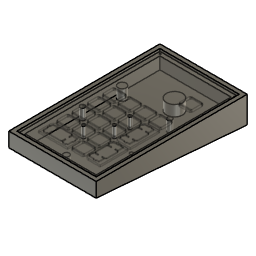
nummerical_case_+_plate (Autodesk Fusion 360 design; units mm, degrees)
Autodesk Fusion 360 part; units mm, degrees
note: some values were not read from the file. Set by a fixed rule: which sketch regions a step uses.
(part 1 of 3)
sketch "ae4adbfa673b0e7a36190fe0facbe4f336e7beb9_switch" plane through (0, 0, 0) normal (0, 0, 1) x (1, 0, 0)
  line L0 (0.0951, 148.071) -> (76.2953, 148.071)
  line L1 (76.2953, 148.071) -> (76.2953, 0.4341)
  line L2 (76.2953, 0.4341) -> (0.0951, 0.4341)
  line L3 (0.0951, 0.4341) -> (0.0951, 148.071)
  line L4 (12.1447, 16.9595) -> (12.1447, 16.3601)
  line L5 (12.1447, 16.3601) -> (11.344, 16.3601)
  line L6 (11.344, 16.3601) -> (11.344, 12.2604)
  line L7 (11.344, 12.2604) -> (10.6192, 12.2604)
  line L8 (10.6192, 12.2604) -> (10.6192, 15.4905)
  line L9 (10.6192, 15.4905) -> (3.8695, 15.4905)
  line L10 (3.8695, 15.4905) -> (3.8695, 12.2604)
  line L11 (3.8695, 12.2604) -> (3.0441, 12.2604)
  line L12 (3.0441, 12.2604) -> (3.0441, 9.4602)
  line L13 (3.0441, 9.4602) -> (3.8696, 9.4602)
  line L14 (3.8695, 9.4602) -> (3.8695, 3.1902)
  line L15 (3.8695, 3.1902) -> (5.5948, 3.1902)
  line L16 (5.5948, 3.1902) -> (5.5948, 1.9899)
  line L17 (5.5948, 1.9899) -> (8.8939, 1.9899)
  line L18 (8.8939, 1.9899) -> (8.8939, 3.1902)
  line L19 (8.8939, 3.1902) -> (10.6192, 3.1902)
  line L20 (10.6192, 3.1902) -> (10.6192, 7.6605)
  line L21 (10.6192, 7.6605) -> (11.344, 7.6605)
  line L22 (11.344, 7.6605) -> (11.344, 3.5609)
  line L23 (11.344, 3.5609) -> (12.1447, 3.5609)
  line L24 (12.1447, 3.5609) -> (12.1447, 2.96)
  line L25 (12.1447, 2.96) -> (26.1441, 2.96)
  line L26 (26.1441, 2.96) -> (26.1441, 3.5609)
  line L27 (26.1441, 3.5609) -> (26.9448, 3.5609)
  line L28 (26.9448, 3.5609) -> (26.9448, 7.6605)
  line L29 (26.9448, 7.6605) -> (27.6696, 7.6605)
  line L30 (27.6696, 7.6605) -> (27.6696, 3.1902)
  line L31 (27.6696, 3.1902) -> (29.3949, 3.1902)
  line L32 (29.3949, 3.1902) -> (29.3949, 1.9899)
  line L33 (29.3949, 1.9899) -> (32.694, 1.9899)
  line L34 (32.694, 1.9899) -> (32.694, 3.1902)
  line L35 (32.694, 3.1902) -> (34.4193, 3.1902)
  line L36 (34.4193, 3.1902) -> (34.4193, 9.4602)
  line L37 (34.4193, 9.4602) -> (35.2447, 9.4602)
  line L38 (35.2447, 9.4602) -> (35.2447, 12.2604)
  line L39 (35.2447, 12.2604) -> (34.4193, 12.2604)
  line L40 (34.4193, 12.2604) -> (34.4193, 15.4905)
  line L41 (34.4193, 15.4905) -> (27.6696, 15.4905)
  line L42 (27.6696, 15.4905) -> (27.6696, 12.2604)
  line L43 (27.6696, 12.2604) -> (26.9448, 12.2604)
  line L44 (26.9448, 12.2604) -> (26.9448, 16.3601)
  line L45 (26.9448, 16.3601) -> (26.1441, 16.3601)
  line L46 (26.1441, 16.3601) -> (26.1441, 16.9595)
  line L47 (26.1441, 16.9595) -> (12.1447, 16.9595)
  line L48 (40.7197, 16.9595) -> (40.7197, 16.3601)
  line L49 (40.7197, 16.3601) -> (39.9189, 16.3601)
  line L50 (39.9189, 16.3601) -> (39.9189, 3.5609)
  line L51 (39.9189, 3.5609) -> (40.7197, 3.5609)
  line L52 (40.7197, 3.5609) -> (40.7197, 2.96)
  line L53 (40.7197, 2.96) -> (54.719, 2.96)
  line L54 (54.719, 2.96) -> (54.719, 3.5609)
  line L55 (54.719, 3.5609) -> (55.5198, 3.5609)
  line L56 (55.5198, 3.5609) -> (55.5198, 16.3601)
  line L57 (55.5198, 16.3601) -> (54.719, 16.3601)
  line L58 (54.719, 16.3601) -> (54.719, 16.9595)
  line L59 (54.719, 16.9595) -> (40.7197, 16.9595)
  line L60 (66.27, 35.585) -> (66.27, 34.7597)
  line L61 (66.27, 34.7597) -> (59.9997, 34.7597)
  line L62 (59.9997, 34.7597) -> (59.9997, 33.0357)
  line L63 (59.9997, 33.0357) -> (58.7996, 33.0357)
  line L64 (58.7996, 33.0357) -> (58.7996, 29.7353)
  line L65 (58.7996, 29.7353) -> (59.9997, 29.7353)
  line L66 (59.9997, 29.7353) -> (59.9997, 28.01)
  line L67 (59.9997, 28.01) -> (64.4701, 28.01)
  line L68 (64.4701, 28.01) -> (64.4701, 27.2852)
  line L69 (64.4701, 27.2852) -> (60.3691, 27.2852)
  line L70 (60.3691, 27.2852) -> (60.3691, 26.4845)
  line L71 (60.3691, 26.4845) -> (59.7697, 26.4845)
  line L72 (59.7697, 26.4845) -> (59.7697, 12.485)
  line L73 (59.7697, 12.485) -> (60.3691, 12.485)
  line L74 (60.3691, 12.485) -> (60.3691, 11.6858)
  line L75 (60.3691, 11.6858) -> (64.4701, 11.6858)
  line L76 (64.4701, 11.6858) -> (64.4701, 10.9595)
  line L77 (64.4701, 10.9595) -> (59.9997, 10.9595)
  line L78 (59.9997, 10.9595) -> (59.9997, 9.2356)
  line L79 (59.9997, 9.2356) -> (58.7996, 9.2356)
  line L80 (58.7996, 9.2356) -> (58.7996, 5.9352)
  line L81 (58.7996, 5.9352) -> (59.9997, 5.9352)
  line L82 (59.9997, 5.9352) -> (59.9997, 4.2099)
  line L83 (59.9997, 4.2099) -> (66.27, 4.2099)
  line L84 (66.27, 4.2099) -> (66.27, 3.3858)
  line L85 (66.27, 3.3858) -> (69.07, 3.3858)
  line L86 (69.07, 3.3858) -> (69.07, 4.2099)
  line L87 (69.07, 4.2099) -> (72.3, 4.2099)
  line L88 (72.3, 4.2099) -> (72.3, 10.9595)
  line L89 (72.3, 10.9595) -> (69.07, 10.9595)
  line L90 (69.07, 10.9595) -> (69.07, 11.6858)
  line L91 (69.07, 11.6858) -> (73.1696, 11.6858)
  line L92 (73.1696, 11.6858) -> (73.1696, 12.485)
  line L93 (73.1696, 12.485) -> (73.769, 12.485)
  line L94 (73.769, 12.485) -> (73.769, 26.4845)
  line L95 (73.769, 26.4845) -> (73.1696, 26.4845)
  line L96 (73.1696, 26.4845) -> (73.1696, 27.2852)
  line L97 (73.1696, 27.2852) -> (69.07, 27.2852)
  line L98 (69.07, 27.2852) -> (69.07, 28.01)
  line L99 (69.07, 28.01) -> (72.3, 28.01)
  line L100 (72.3, 28.01) -> (72.3, 34.7597)
  line L101 (72.3, 34.7597) -> (69.07, 34.7597)
  line L102 (69.07, 34.7597) -> (69.07, 35.585)
  line L103 (69.07, 35.585) -> (66.27, 35.585)
  line L104 (2.6197, 36.0094) -> (2.6197, 35.4101)
  line L105 (2.6197, 35.4101) -> (1.819, 35.4101)
  line L106 (1.819, 35.4101) -> (1.819, 22.6109)
  line L107 (1.819, 22.6109) -> (2.6197, 22.6109)
  line L108 (2.6197, 22.6109) -> (2.6197, 22.01)
  line L109 (2.6197, 22.01) -> (16.6192, 22.01)
  line L110 (16.6192, 22.01) -> (16.6192, 22.6109)
  line L111 (16.6192, 22.6109) -> (17.4198, 22.6109)
  line L112 (17.4198, 22.6109) -> (17.4198, 35.4101)
  line L113 (17.4198, 35.4101) -> (16.6192, 35.4101)
  line L114 (16.6192, 35.4101) -> (16.6192, 36.0094)
  line L115 (16.6192, 36.0094) -> (2.6196, 36.0094)
  line L116 (21.6697, 36.0094) -> (21.6697, 35.4101)
  line L117 (21.6697, 35.4101) -> (20.869, 35.4101)
  line L118 (20.869, 35.4101) -> (20.869, 22.6109)
  line L119 (20.869, 22.6109) -> (21.6697, 22.6109)
  line L120 (21.6697, 22.6109) -> (21.6697, 22.01)
  line L121 (21.6697, 22.01) -> (35.669, 22.01)
  line L122 (35.669, 22.01) -> (35.669, 22.6109)
  line L123 (35.669, 22.6109) -> (36.4698, 22.6109)
  line L124 (36.4698, 22.6109) -> (36.4698, 35.4101)
  line L125 (36.4698, 35.4101) -> (35.669, 35.4101)
  line L126 (35.669, 35.4101) -> (35.669, 36.0094)
  line L127 (35.669, 36.0094) -> (21.6697, 36.0094)
  line L128 (40.7197, 36.0094) -> (40.7197, 35.4101)
  line L129 (40.7197, 35.4101) -> (39.9189, 35.4101)
  line L130 (39.9189, 35.4101) -> (39.9189, 22.6109)
  line L131 (39.9189, 22.6109) -> (40.7197, 22.6109)
  line L132 (40.7197, 22.6109) -> (40.7197, 22.01)
  line L133 (40.7197, 22.01) -> (54.719, 22.01)
  line L134 (54.719, 22.01) -> (54.719, 22.6109)
  line L135 (54.719, 22.6109) -> (55.5198, 22.6109)
  line L136 (55.5198, 22.6109) -> (55.5198, 35.4101)
  line L137 (55.5198, 35.4101) -> (54.719, 35.4101)
  line L138 (54.719, 35.4101) -> (54.719, 36.0094)
  line L139 (54.719, 36.0094) -> (40.7197, 36.0094)
  line L140 (2.6197, 55.0594) -> (2.6197, 54.4601)
  line L141 (2.6197, 54.4601) -> (1.819, 54.4601)
  line L142 (1.819, 54.4601) -> (1.819, 41.6609)
  line L143 (1.819, 41.6609) -> (2.6197, 41.6609)
  line L144 (2.6197, 41.6609) -> (2.6197, 41.0602)
  line L145 (2.6197, 41.0602) -> (16.6192, 41.0602)
  line L146 (16.6192, 41.0602) -> (16.6192, 41.6609)
  line L147 (16.6192, 41.6609) -> (17.4198, 41.6609)
  line L148 (17.4198, 41.6609) -> (17.4198, 54.4601)
  line L149 (17.4198, 54.4601) -> (16.6192, 54.4601)
  line L150 (16.6192, 54.4601) -> (16.6192, 55.0594)
  line L151 (16.6192, 55.0594) -> (2.6196, 55.0594)
  line L152 (21.6697, 55.0594) -> (21.6697, 54.4601)
  line L153 (21.6697, 54.4601) -> (20.869, 54.4601)
  line L154 (20.869, 54.4601) -> (20.869, 41.6609)
  line L155 (20.869, 41.6609) -> (21.6697, 41.6609)
  line L156 (21.6697, 41.6609) -> (21.6697, 41.0602)
  line L157 (21.6697, 41.0602) -> (35.669, 41.0602)
  line L158 (35.669, 41.0602) -> (35.669, 41.6609)
  line L159 (35.669, 41.6609) -> (36.4698, 41.6609)
  line L160 (36.4698, 41.6609) -> (36.4698, 54.4601)
  line L161 (36.4698, 54.4601) -> (35.669, 54.4601)
  line L162 (35.669, 54.4601) -> (35.669, 55.0594)
  line L163 (35.669, 55.0594) -> (21.6697, 55.0594)
  line L164 (40.7197, 55.0594) -> (40.7197, 54.4601)
  line L165 (40.7197, 54.4601) -> (39.9189, 54.4601)
  line L166 (39.9189, 54.4601) -> (39.9189, 41.6609)
  line L167 (39.9189, 41.6609) -> (40.7197, 41.6609)
  line L168 (40.7197, 41.6609) -> (40.7197, 41.0602)
  line L169 (40.7197, 41.0602) -> (54.719, 41.0602)
  line L170 (54.719, 41.0602) -> (54.719, 41.6609)
  line L171 (54.719, 41.6609) -> (55.5198, 41.6609)
  line L172 (55.5198, 41.6609) -> (55.5198, 54.4601)
  line L173 (55.5198, 54.4601) -> (54.719, 54.4601)
  line L174 (54.719, 54.4601) -> (54.719, 55.0594)
  line L175 (54.719, 55.0594) -> (40.7197, 55.0594)
  line L176 (66.27, 73.685) -> (66.27, 72.8595)
  line L177 (66.27, 72.8595) -> (59.9997, 72.8595)
  line L178 (59.9997, 72.8595) -> (59.9997, 71.1359)
  line L179 (59.9997, 71.1359) -> (58.7996, 71.1359)
  line L180 (58.7996, 71.1359) -> (58.7996, 67.8353)
  line L181 (58.7996, 67.8353) -> (59.9997, 67.8353)
  line L182 (59.9997, 67.8353) -> (59.9997, 66.1098)
  line L183 (59.9997, 66.1098) -> (64.4701, 66.1098)
  line L184 (64.4701, 66.1098) -> (64.4701, 65.3852)
  line L185 (64.4701, 65.3852) -> (60.3691, 65.3852)
  line L186 (60.3691, 65.3852) -> (60.3691, 64.5844)
  line L187 (60.3691, 64.5844) -> (59.7697, 64.5844)
  line L188 (59.7697, 64.5844) -> (59.7697, 50.5852)
  line L189 (59.7697, 50.5852) -> (60.3691, 50.5852)
  line L190 (60.3691, 50.5852) -> (60.3691, 49.7858)
  line L191 (60.3691, 49.7858) -> (64.4701, 49.7858)
  line L192 (64.4701, 49.7858) -> (64.4701, 49.0594)
  line L193 (64.4701, 49.0594) -> (59.9997, 49.0594)
  line L194 (59.9997, 49.0594) -> (59.9997, 47.3357)
  line L195 (59.9997, 47.3357) -> (58.7996, 47.3357)
  line L196 (58.7996, 47.3357) -> (58.7996, 44.0351)
  line L197 (58.7996, 44.0351) -> (59.9997, 44.0351)
  line L198 (59.9997, 44.0351) -> (59.9997, 42.31)
  line L199 (59.9997, 42.31) -> (66.27, 42.31)
  line L200 (66.27, 42.31) -> (66.27, 41.486)
  line L201 (66.27, 41.486) -> (69.07, 41.486)
  line L202 (69.07, 41.486) -> (69.07, 42.31)
  line L203 (69.07, 42.31) -> (72.3, 42.31)
  line L204 (72.3, 42.31) -> (72.3, 49.0594)
  line L205 (72.3, 49.0594) -> (69.07, 49.0594)
  line L206 (69.07, 49.0594) -> (69.07, 49.7858)
  line L207 (69.07, 49.7858) -> (73.1696, 49.7858)
  line L208 (73.1696, 49.7858) -> (73.1696, 50.5852)
  line L209 (73.1696, 50.5852) -> (73.769, 50.5852)
  line L210 (73.769, 50.5852) -> (73.769, 64.5844)
  line L211 (73.769, 64.5844) -> (73.1696, 64.5844)
  line L212 (73.1696, 64.5844) -> (73.1696, 65.3852)
  line L213 (73.1696, 65.3852) -> (69.07, 65.3852)
  line L214 (69.07, 65.3852) -> (69.07, 66.1098)
  line L215 (69.07, 66.1098) -> (72.3, 66.1098)
  line L216 (72.3, 66.1098) -> (72.3, 72.8595)
  line L217 (72.3, 72.8595) -> (69.07, 72.8595)
  line L218 (69.07, 72.8595) -> (69.07, 73.685)
  line L219 (69.07, 73.685) -> (66.27, 73.685)
  line L220 (2.6197, 74.1094) -> (2.6197, 73.5101)
  line L221 (2.6197, 73.5101) -> (1.819, 73.5101)
  line L222 (1.819, 73.5101) -> (1.819, 60.7109)
  line L223 (1.819, 60.7109) -> (2.6197, 60.7109)
  line L224 (2.6197, 60.7109) -> (2.6197, 60.1102)
  line L225 (2.6197, 60.1102) -> (16.6192, 60.1102)
  line L226 (16.6192, 60.1102) -> (16.6192, 60.7109)
  line L227 (16.6192, 60.7109) -> (17.4198, 60.7109)
  line L228 (17.4198, 60.7109) -> (17.4198, 73.5101)
  line L229 (17.4198, 73.5101) -> (16.6192, 73.5101)
  line L230 (16.6192, 73.5101) -> (16.6192, 74.1094)
  line L231 (16.6192, 74.1094) -> (2.6196, 74.1094)
  line L232 (21.6697, 74.1094) -> (21.6697, 73.5101)
  line L233 (21.6697, 73.5101) -> (20.869, 73.5101)
  line L234 (20.869, 73.5101) -> (20.869, 60.7109)
  line L235 (20.869, 60.7109) -> (21.6697, 60.7109)
  line L236 (21.6697, 60.7109) -> (21.6697, 60.1102)
  line L237 (21.6697, 60.1102) -> (35.669, 60.1102)
  line L238 (35.669, 60.1102) -> (35.669, 60.7109)
  line L239 (35.669, 60.7109) -> (36.4698, 60.7109)
  line L240 (36.4698, 60.7109) -> (36.4698, 73.5101)
  line L241 (36.4698, 73.5101) -> (35.669, 73.5101)
  line L242 (35.669, 73.5101) -> (35.669, 74.1094)
  line L243 (35.669, 74.1094) -> (21.6697, 74.1094)
  line L244 (40.7197, 74.1094) -> (40.7197, 73.5101)
  line L245 (40.7197, 73.5101) -> (39.9189, 73.5101)
  line L246 (39.9189, 73.5101) -> (39.9189, 60.7109)
  line L247 (39.9189, 60.7109) -> (40.7197, 60.7109)
  line L248 (40.7197, 60.7109) -> (40.7197, 60.1102)
  line L249 (40.7197, 60.1102) -> (54.719, 60.1102)
  line L250 (54.719, 60.1102) -> (54.719, 60.7109)
  line L251 (54.719, 60.7109) -> (55.5198, 60.7109)
  line L252 (55.5198, 60.7109) -> (55.5198, 73.5101)
  line L253 (55.5198, 73.5101) -> (54.719, 73.5101)
  line L254 (54.719, 73.5101) -> (54.719, 74.1094)
  line L255 (54.719, 74.1094) -> (40.7197, 74.1094)
  line L256 (2.6197, 93.1594) -> (2.6197, 92.5601)
  line L257 (2.6197, 92.5601) -> (1.819, 92.5601)
  line L258 (1.819, 92.5601) -> (1.819, 79.7609)
  line L259 (1.819, 79.7609) -> (2.6197, 79.7609)
  line L260 (2.6197, 79.7609) -> (2.6197, 79.1602)
  line L261 (2.6197, 79.1602) -> (16.6192, 79.1602)
  line L262 (16.6192, 79.1602) -> (16.6192, 79.7609)
  line L263 (16.6192, 79.7609) -> (17.4198, 79.7609)
  line L264 (17.4198, 79.7609) -> (17.4198, 92.5601)
  line L265 (17.4198, 92.5601) -> (16.6192, 92.5601)
  line L266 (16.6192, 92.5601) -> (16.6192, 93.1594)
  line L267 (16.6192, 93.1594) -> (2.6196, 93.1594)
  line L268 (21.6697, 93.1594) -> (21.6697, 92.5601)
  line L269 (21.6697, 92.5601) -> (20.869, 92.5601)
  line L270 (20.869, 92.5601) -> (20.869, 79.7609)
  line L271 (20.869, 79.7609) -> (21.6697, 79.7609)
  line L272 (21.6697, 79.7609) -> (21.6697, 79.1602)
  line L273 (21.6697, 79.1602) -> (35.669, 79.1602)
  line L274 (35.669, 79.1602) -> (35.669, 79.7609)
  line L275 (35.669, 79.7609) -> (36.4698, 79.7609)
  line L276 (36.4698, 79.7609) -> (36.4698, 92.5601)
  line L277 (36.4698, 92.5601) -> (35.669, 92.5601)
  line L278 (35.669, 92.5601) -> (35.669, 93.1594)
  line L279 (35.669, 93.1594) -> (21.6697, 93.1594)
  line L280 (40.7197, 93.1594) -> (40.7197, 92.5601)
  line L281 (40.7197, 92.5601) -> (39.9189, 92.5601)
  line L282 (39.9189, 92.5601) -> (39.9189, 79.7609)
  line L283 (39.9189, 79.7609) -> (40.7197, 79.7609)
  line L284 (40.7197, 79.7609) -> (40.7197, 79.1602)
  line L285 (40.7197, 79.1602) -> (54.719, 79.1602)
  line L286 (54.719, 79.1602) -> (54.719, 79.7609)
  line L287 (54.719, 79.7609) -> (55.5198, 79.7609)
  line L288 (55.5198, 79.7609) -> (55.5198, 92.5601)
  line L289 (55.5198, 92.5601) -> (54.719, 92.5601)
  line L290 (54.719, 92.5601) -> (54.719, 93.1594)
  line L291 (54.719, 93.1594) -> (40.7197, 93.1594)
  line L292 (59.7697, 93.1594) -> (59.7697, 92.5601)
  line L293 (59.7697, 92.5601) -> (58.9689, 92.5601)
  line L294 (58.9689, 92.5601) -> (58.9689, 79.7609)
  line L295 (58.9689, 79.7609) -> (59.7697, 79.7609)
  line L296 (59.7697, 79.7609) -> (59.7697, 79.1602)
  line L297 (59.7697, 79.1602) -> (73.769, 79.1602)
  line L298 (73.769, 79.1602) -> (73.769, 79.7609)
  line L299 (73.769, 79.7609) -> (74.5698, 79.7609)
  line L300 (74.5698, 79.7609) -> (74.5698, 92.5601)
  line L301 (74.5698, 92.5601) -> (73.769, 92.5601)
  line L302 (73.769, 92.5601) -> (73.769, 93.1594)
  line L303 (73.769, 93.1594) -> (59.7697, 93.1594)
  line L304 (59.7697, 131.259) -> (59.7697, 130.66)
  line L305 (59.7697, 130.66) -> (58.9689, 130.66)
  line L306 (58.9689, 130.66) -> (58.9689, 117.861)
  line L307 (58.9689, 117.861) -> (59.7697, 117.861)
  line L308 (59.7697, 117.861) -> (59.7697, 117.26)
  line L309 (59.7697, 117.26) -> (73.769, 117.26)
  line L310 (73.769, 117.26) -> (73.769, 117.861)
  line L311 (73.769, 117.861) -> (74.5698, 117.861)
  line L312 (74.5698, 117.861) -> (74.5698, 130.66)
  line L313 (74.5698, 130.66) -> (73.769, 130.66)
  line L314 (73.769, 130.66) -> (73.769, 131.259)
  line L315 (73.769, 131.259) -> (59.7697, 131.259)
extrude "Extrude1" add sketch "ae4adbfa673b0e7a36190fe0facbe4f336e7beb9_switch" along normal blind 1 makes body 1
extrude "Extrude2" add 1 faces at (26.9112, 123.9635, 0) along direction (0, 0, -1) blind 2 separate body on bodies 1 makes body 2
extrude "Extrude3" cut 1 faces at (69.1026, 131.259, -0.6667) along direction (0, 1, 0) blind 1 on bodies 2 bodies 2
extrude "Extrude4" cut 4 faces at (69.1026, 93.1594, -0.6667) (50.0526, 93.1594, -0.6667) (31.0026, 93.1594, -0.6667) (11.9527, 93.1594, -0.6667) along direction (0, 1, 0) blind 1 on bodies 2 bodies 2
extrude "Extrude5" cut 3 faces at (50.0526, 74.1094, -0.6667) (31.0026, 74.1094, -0.6667) (11.9527, 74.1094, -0.6667) along direction (0, 1, 0) blind 1 on bodies 2 bodies 2
extrude "Extrude6" cut 3 faces at (50.0526, 55.0594, -0.6667) (31.0026, 55.0594, -0.6667) (11.9527, 55.0594, -0.6667) along direction (0, 1, 0) blind 1 on bodies 2 bodies 2
extrude "Extrude7" cut 3 faces at (50.0526, 36.0094, -0.6667) (31.0026, 36.0094, -0.6667) (11.9527, 36.0094, -0.6667) along direction (0, 1, 0) blind 1 on bodies 2 bodies 2
extrude "Extrude8" cut 2 faces at (50.0526, 16.9595, -0.6667) (21.4776, 16.9595, -0.6667) along direction (0, 1, 0) blind 1 on bodies 2 bodies 2
extrude "Extrude9" cut 2 faces at (73.769, 55.2516, -0.6667) (73.769, 17.1515, -0.6667) along direction (1, 0, 0) blind 1 on bodies 2 bodies 2
extrude "Extrude10" cut 2 faces at (59.7697, 59.918, -0.6667) (59.7697, 21.818, -0.6667) along direction (-1, 0, 0) blind 1 on bodies 2 bodies 2
extrude "Extrude11" cut 2 faces at (45.3861, 2.96, -0.6667) (16.8112, 2.96, -0.6667) along direction (0, -1, 0) blind 1 on bodies 2 bodies 2
extrude "Extrude12" cut 3 faces at (45.3861, 79.1602, -0.6667) (26.3361, 79.1602, -0.6667) (7.2862, 79.1602, -0.6667) along direction (0, -1, 0) blind 1 on bodies 2 bodies 2
extrude "Extrude13" cut 1 faces at (64.4361, 79.1602, -0.6667) along direction (0, -1, 0) blind 1 on bodies 2 bodies 2
extrude "Extrude14" cut 3 faces at (45.3861, 60.1102, -0.6667) (26.3361, 60.1102, -0.6667) (7.2862, 60.1102, -0.6667) along direction (0, -1, 0) blind 1 on bodies 2 bodies 2
extrude "Extrude15" cut 3 faces at (7.2862, 41.0602, -0.6667) (26.3361, 41.0602, -0.6667) (45.3861, 41.0602, -0.6667) along direction (0, -1, 0) blind 1 on bodies 2 bodies 2
extrude "Extrude16" cut 3 faces at (45.3861, 22.01, -0.6667) (26.3361, 22.01, -0.6667) (7.2862, 22.01, -0.6667) along direction (0, -1, 0) blind 1 on bodies 2 bodies 2
extrude "Extrude17" cut 1 faces at (64.4361, 117.26, -0.6667) along direction (0, -1, 0) blind 1 on bodies 2 bodies 2
sketch "Sketch2" plane through (0, 0, -2) normal (0, 0, -1) x (1, 0, 0)
  line L0 (21.6697, -60.7109) -> (21.6697, -59.1102)
  line L1 (21.6697, -59.1102) -> (35.669, -59.1102)
  line L2 (35.669, -59.1102) -> (35.669, -60.7109)
  line L3 (35.669, -60.7109) -> (36.4698, -60.7109)
  line L4 (36.4698, -60.7109) -> (36.4698, -73.5101)
  line L5 (36.4698, -73.5101) -> (35.669, -73.5101)
  line L6 (35.669, -73.5101) -> (35.669, -75.1094)
  line L7 (35.669, -75.1094) -> (21.6697, -75.1094)
  line L8 (21.6697, -75.1094) -> (21.6697, -73.5101)
  line L9 (21.6697, -73.5101) -> (20.869, -73.5101)
  line L10 (20.869, -73.5101) -> (20.869, -60.7109)
  line L11 (20.869, -60.7109) -> (21.6697, -60.7109)
  line L12 (60.3691, -26.4845) -> (58.7697, -26.4845)
  line L13 (58.7697, -26.4845) -> (58.7697, -12.485)
  line L14 (58.7697, -12.485) -> (60.3691, -12.485)
  line L15 (60.3691, -12.485) -> (60.3691, -11.6858)
  line L16 (60.3691, -11.6858) -> (64.4701, -11.6858)
  line L17 (64.4701, -11.6858) -> (64.4701, -10.9595)
  line L18 (64.4701, -10.9595) -> (59.9997, -10.9595)
  line L19 (59.9997, -10.9595) -> (59.9997, -9.2356)
  line L20 (59.9997, -9.2356) -> (58.7996, -9.2356)
  line L21 (58.7996, -9.2356) -> (58.7996, -5.9352)
  line L22 (58.7996, -5.9352) -> (59.9997, -5.9352)
  line L23 (59.9997, -5.9352) -> (59.9997, -4.2099)
  line L24 (59.9997, -4.2099) -> (66.27, -4.2099)
  line L25 (66.27, -4.2099) -> (66.27, -3.3858)
  line L26 (66.27, -3.3858) -> (69.07, -3.3858)
  line L27 (69.07, -3.3858) -> (69.07, -4.2099)
  line L28 (69.07, -4.2099) -> (72.3, -4.2099)
  line L29 (72.3, -4.2099) -> (72.3, -10.9595)
  line L30 (72.3, -10.9595) -> (69.07, -10.9595)
  line L31 (69.07, -10.9595) -> (69.07, -11.6858)
  line L32 (69.07, -11.6858) -> (73.1696, -11.6858)
  line L33 (73.1696, -11.6858) -> (73.1696, -12.485)
  line L34 (73.1696, -12.485) -> (74.769, -12.485)
  line L35 (74.769, -12.485) -> (74.769, -26.4845)
  line L36 (74.769, -26.4845) -> (73.1696, -26.4845)
  line L37 (73.1696, -26.4845) -> (73.1696, -27.2852)
  line L38 (73.1696, -27.2852) -> (69.07, -27.2852)
  line L39 (69.07, -27.2852) -> (69.07, -28.01)
  line L40 (69.07, -28.01) -> (72.3, -28.01)
  line L41 (72.3, -28.01) -> (72.3, -34.7597)
  line L42 (72.3, -34.7597) -> (69.07, -34.7597)
  line L43 (69.07, -34.7597) -> (69.07, -35.585)
  line L44 (69.07, -35.585) -> (66.27, -35.585)
  line L45 (66.27, -35.585) -> (66.27, -34.7597)
  line L46 (66.27, -34.7597) -> (59.9997, -34.7597)
  line L47 (59.9997, -34.7597) -> (59.9997, -33.0357)
  line L48 (59.9997, -33.0357) -> (58.7996, -33.0357)
  line L49 (58.7996, -33.0357) -> (58.7996, -29.7353)
  line L50 (58.7996, -29.7353) -> (59.9997, -29.7353)
  line L51 (59.9997, -29.7353) -> (59.9997, -28.01)
  line L52 (59.9997, -28.01) -> (64.4701, -28.01)
  line L53 (64.4701, -28.01) -> (64.4701, -27.2852)
  line L54 (64.4701, -27.2852) -> (60.3691, -27.2852)
  line L55 (60.3691, -27.2852) -> (60.3691, -26.4845)
  line L56 (21.6697, -79.7609) -> (21.6697, -78.1602)
  line L57 (21.6697, -78.1602) -> (35.669, -78.1602)
  line L58 (35.669, -78.1602) -> (35.669, -79.7609)
  line L59 (35.669, -79.7609) -> (36.4698, -79.7609)
  line L60 (36.4698, -79.7609) -> (36.4698, -92.5601)
  line L61 (36.4698, -92.5601) -> (35.669, -92.5601)
  line L62 (35.669, -92.5601) -> (35.669, -94.1594)
  line L63 (35.669, -94.1594) -> (21.6697, -94.1594)
  line L64 (21.6697, -94.1594) -> (21.6697, -92.5601)
  line L65 (21.6697, -92.5601) -> (20.869, -92.5601)
  line L66 (20.869, -92.5601) -> (20.869, -79.7609)
  line L67 (20.869, -79.7609) -> (21.6697, -79.7609)
  line L68 (59.7697, -117.861) -> (59.7697, -116.26)
  line L69 (59.7697, -116.26) -> (73.769, -116.26)
  line L70 (73.769, -116.26) -> (73.769, -117.861)
  line L71 (73.769, -117.861) -> (74.5698, -117.861)
  line L72 (74.5698, -117.861) -> (74.5698, -130.66)
  line L73 (74.5698, -130.66) -> (73.769, -130.66)
  line L74 (73.769, -130.66) -> (73.769, -132.259)
  line L75 (73.769, -132.259) -> (59.7697, -132.259)
  line L76 (59.7697, -132.259) -> (59.7697, -130.66)
  line L77 (59.7697, -130.66) -> (58.9689, -130.66)
  line L78 (58.9689, -130.66) -> (58.9689, -117.861)
  line L79 (58.9689, -117.861) -> (59.7697, -117.861)
  line L80 (60.3691, -64.5844) -> (58.7697, -64.5844)
  line L81 (58.7697, -64.5844) -> (58.7697, -50.5852)
  line L82 (58.7697, -50.5852) -> (60.3691, -50.5852)
  line L83 (60.3691, -50.5852) -> (60.3691, -49.7858)
  line L84 (60.3691, -49.7858) -> (64.4701, -49.7858)
  line L85 (64.4701, -49.7858) -> (64.4701, -49.0594)
  line L86 (64.4701, -49.0594) -> (59.9997, -49.0594)
  line L87 (59.9997, -49.0594) -> (59.9997, -47.3357)
  line L88 (59.9997, -47.3357) -> (58.7996, -47.3357)
  line L89 (58.7996, -47.3357) -> (58.7996, -44.0351)
  line L90 (58.7996, -44.0351) -> (59.9997, -44.0351)
  line L91 (59.9997, -44.0351) -> (59.9997, -42.31)
  line L92 (59.9997, -42.31) -> (66.27, -42.31)
  line L93 (66.27, -42.31) -> (66.27, -41.486)
  line L94 (66.27, -41.486) -> (69.07, -41.486)
  line L95 (69.07, -41.486) -> (69.07, -42.31)
  line L96 (69.07, -42.31) -> (72.3, -42.31)
  line L97 (72.3, -42.31) -> (72.3, -49.0594)
  line L98 (72.3, -49.0594) -> (69.07, -49.0594)
  line L99 (69.07, -49.0594) -> (69.07, -49.7858)
  line L100 (69.07, -49.7858) -> (73.1696, -49.7858)
  line L101 (73.1696, -49.7858) -> (73.1696, -50.5852)
  line L102 (73.1696, -50.5852) -> (74.769, -50.5852)
  line L103 (74.769, -50.5852) -> (74.769, -64.5844)
  line L104 (74.769, -64.5844) -> (73.1696, -64.5844)
  line L105 (73.1696, -64.5844) -> (73.1696, -65.3852)
  line L106 (73.1696, -65.3852) -> (69.07, -65.3852)
  line L107 (69.07, -65.3852) -> (69.07, -66.1098)
  line L108 (69.07, -66.1098) -> (72.3, -66.1098)
  line L109 (72.3, -66.1098) -> (72.3, -72.8595)
  line L110 (72.3, -72.8595) -> (69.07, -72.8595)
  line L111 (69.07, -72.8595) -> (69.07, -73.685)
  line L112 (69.07, -73.685) -> (66.27, -73.685)
  line L113 (66.27, -73.685) -> (66.27, -72.8595)
  line L114 (66.27, -72.8595) -> (59.9997, -72.8595)
  line L115 (59.9997, -72.8595) -> (59.9997, -71.1359)
  line L116 (59.9997, -71.1359) -> (58.7996, -71.1359)
  line L117 (58.7996, -71.1359) -> (58.7996, -67.8353)
  line L118 (58.7996, -67.8353) -> (59.9997, -67.8353)
  line L119 (59.9997, -67.8353) -> (59.9997, -66.1098)
  line L120 (59.9997, -66.1098) -> (64.4701, -66.1098)
  line L121 (64.4701, -66.1098) -> (64.4701, -65.3852)
  line L122 (64.4701, -65.3852) -> (60.3691, -65.3852)
  line L123 (60.3691, -65.3852) -> (60.3691, -64.5844)
  line L124 (2.6197, -60.7109) -> (2.6197, -59.1102)
  line L125 (2.6197, -59.1102) -> (16.6192, -59.1102)
  line L126 (16.6192, -59.1102) -> (16.6192, -60.7109)
  line L127 (16.6192, -60.7109) -> (17.4198, -60.7109)
  line L128 (17.4198, -60.7109) -> (17.4198, -73.5101)
  line L129 (17.4198, -73.5101) -> (16.6192, -73.5101)
  line L130 (16.6192, -73.5101) -> (16.6192, -75.1094)
  line L131 (16.6192, -75.1094) -> (2.6196, -75.1094)
  line L132 (2.6197, -75.1094) -> (2.6197, -73.5101)
  line L133 (2.6197, -73.5101) -> (1.819, -73.5101)
  line L134 (1.819, -73.5101) -> (1.819, -60.7109)
  line L135 (1.819, -60.7109) -> (2.6197, -60.7109)
  line L136 (59.7697, -79.7609) -> (59.7697, -78.1602)
  line L137 (59.7697, -78.1602) -> (73.769, -78.1602)
  line L138 (73.769, -78.1602) -> (73.769, -79.7609)
  line L139 (73.769, -79.7609) -> (74.5698, -79.7609)
  line L140 (74.5698, -79.7609) -> (74.5698, -92.5601)
  line L141 (74.5698, -92.5601) -> (73.769, -92.5601)
  line L142 (73.769, -92.5601) -> (73.769, -94.1594)
  line L143 (73.769, -94.1594) -> (59.7697, -94.1594)
  line L144 (59.7697, -94.1594) -> (59.7697, -92.5601)
  line L145 (59.7697, -92.5601) -> (58.9689, -92.5601)
  line L146 (58.9689, -92.5601) -> (58.9689, -79.7609)
  line L147 (58.9689, -79.7609) -> (59.7697, -79.7609)
  line L148 (40.7197, -79.7609) -> (40.7197, -78.1602)
  line L149 (40.7197, -78.1602) -> (54.719, -78.1602)
  line L150 (54.719, -78.1602) -> (54.719, -79.7609)
  line L151 (54.719, -79.7609) -> (55.5198, -79.7609)
  line L152 (55.5198, -79.7609) -> (55.5198, -92.5601)
  line L153 (55.5198, -92.5601) -> (54.719, -92.5601)
  line L154 (54.719, -92.5601) -> (54.719, -94.1594)
  line L155 (54.719, -94.1594) -> (40.7197, -94.1594)
  line L156 (40.7197, -94.1594) -> (40.7197, -92.5601)
  line L157 (40.7197, -92.5601) -> (39.9189, -92.5601)
  line L158 (39.9189, -92.5601) -> (39.9189, -79.7609)
  line L159 (39.9189, -79.7609) -> (40.7197, -79.7609)
  line L160 (2.6197, -22.6109) -> (2.6197, -21.01)
  line L161 (2.6197, -21.01) -> (16.6192, -21.01)
  line L162 (16.6192, -21.01) -> (16.6192, -22.6109)
  line L163 (16.6192, -22.6109) -> (17.4198, -22.6109)
  line L164 (17.4198, -22.6109) -> (17.4198, -35.4101)
  line L165 (17.4198, -35.4101) -> (16.6192, -35.4101)
  line L166 (16.6192, -35.4101) -> (16.6192, -37.0094)
  line L167 (16.6192, -37.0094) -> (2.6196, -37.0094)
  line L168 (2.6197, -37.0094) -> (2.6197, -35.4101)
  line L169 (2.6197, -35.4101) -> (1.819, -35.4101)
  line L170 (1.819, -35.4101) -> (1.819, -22.6109)
  line L171 (1.819, -22.6109) -> (2.6197, -22.6109)
  line L172 (2.6197, -41.6609) -> (2.6197, -40.0602)
  line L173 (2.6197, -40.0602) -> (16.6192, -40.0602)
  line L174 (16.6192, -40.0602) -> (16.6192, -41.6609)
  line L175 (16.6192, -41.6609) -> (17.4198, -41.6609)
  line L176 (17.4198, -41.6609) -> (17.4198, -54.4601)
  line L177 (17.4198, -54.4601) -> (16.6192, -54.4601)
  line L178 (16.6192, -54.4601) -> (16.6192, -56.0594)
  line L179 (16.6192, -56.0594) -> (2.6196, -56.0594)
  line L180 (2.6197, -56.0594) -> (2.6197, -54.4601)
  line L181 (2.6197, -54.4601) -> (1.819, -54.4601)
  line L182 (1.819, -54.4601) -> (1.819, -41.6609)
  line L183 (1.819, -41.6609) -> (2.6197, -41.6609)
  line L184 (21.6697, -41.6609) -> (21.6697, -40.0602)
  line L185 (21.6697, -40.0602) -> (35.669, -40.0602)
  line L186 (35.669, -40.0602) -> (35.669, -41.6609)
  line L187 (35.669, -41.6609) -> (36.4698, -41.6609)
  line L188 (36.4698, -41.6609) -> (36.4698, -54.4601)
  line L189 (36.4698, -54.4601) -> (35.669, -54.4601)
  line L190 (35.669, -54.4601) -> (35.669, -56.0594)
  line L191 (35.669, -56.0594) -> (21.6697, -56.0594)
  line L192 (21.6697, -56.0594) -> (21.6697, -54.4601)
  line L193 (21.6697, -54.4601) -> (20.869, -54.4601)
  line L194 (20.869, -54.4601) -> (20.869, -41.6609)
  line L195 (20.869, -41.6609) -> (21.6697, -41.6609)
  line L196 (40.7197, -60.7109) -> (40.7197, -59.1102)
  line L197 (40.7197, -59.1102) -> (54.719, -59.1102)
  line L198 (54.719, -59.1102) -> (54.719, -60.7109)
  line L199 (54.719, -60.7109) -> (55.5198, -60.7109)
  line L200 (55.5198, -60.7109) -> (55.5198, -73.5101)
  line L201 (55.5198, -73.5101) -> (54.719, -73.5101)
  line L202 (54.719, -73.5101) -> (54.719, -75.1094)
  line L203 (54.719, -75.1094) -> (40.7197, -75.1094)
  line L204 (40.7197, -75.1094) -> (40.7197, -73.5101)
  line L205 (40.7197, -73.5101) -> (39.9189, -73.5101)
  line L206 (39.9189, -73.5101) -> (39.9189, -60.7109)
  line L207 (39.9189, -60.7109) -> (40.7197, -60.7109)
  line L208 (12.1447, -3.5609) -> (12.1447, -1.96)
  line L209 (12.1447, -1.96) -> (26.1441, -1.96)
  line L210 (26.1441, -1.96) -> (26.1441, -3.5609)
  line L211 (26.1441, -3.5609) -> (26.9448, -3.5609)
  line L212 (26.9448, -3.5609) -> (26.9448, -7.6605)
  line L213 (26.9448, -7.6605) -> (27.6696, -7.6605)
  line L214 (27.6696, -7.6605) -> (27.6696, -3.1902)
  line L215 (27.6696, -3.1902) -> (29.3949, -3.1902)
  line L216 (29.3949, -3.1902) -> (29.3949, -1.9899)
  line L217 (29.3949, -1.9899) -> (32.694, -1.9899)
  line L218 (32.694, -1.9899) -> (32.694, -3.1902)
  line L219 (32.694, -3.1902) -> (34.4193, -3.1902)
  line L220 (34.4193, -3.1902) -> (34.4193, -9.4602)
  line L221 (34.4193, -9.4602) -> (35.2447, -9.4602)
  line L222 (35.2447, -9.4602) -> (35.2447, -12.2604)
  line L223 (35.2447, -12.2604) -> (34.4193, -12.2604)
  line L224 (34.4193, -12.2604) -> (34.4193, -15.4905)
  line L225 (34.4193, -15.4905) -> (27.6696, -15.4905)
  line L226 (27.6696, -15.4905) -> (27.6696, -12.2604)
  line L227 (27.6696, -12.2604) -> (26.9448, -12.2604)
  line L228 (26.9448, -12.2604) -> (26.9448, -16.3601)
  line L229 (26.9448, -16.3601) -> (26.1441, -16.3601)
  line L230 (26.1441, -16.3601) -> (26.1441, -17.9595)
  line L231 (26.1441, -17.9595) -> (12.1447, -17.9595)
  line L232 (12.1447, -17.9595) -> (12.1447, -16.3601)
  line L233 (12.1447, -16.3601) -> (11.344, -16.3601)
  line L234 (11.344, -16.3601) -> (11.344, -12.2604)
  line L235 (11.344, -12.2604) -> (10.6192, -12.2604)
  line L236 (10.6192, -12.2604) -> (10.6192, -15.4905)
  line L237 (10.6192, -15.4905) -> (3.8695, -15.4905)
  line L238 (3.8695, -15.4905) -> (3.8695, -12.2604)
  line L239 (3.8695, -12.2604) -> (3.0441, -12.2604)
  line L240 (3.0441, -12.2604) -> (3.0441, -9.4602)
  line L241 (3.0441, -9.4602) -> (3.8695, -9.4602)
  line L242 (3.8695, -9.4602) -> (3.8695, -3.1902)
  line L243 (3.8695, -3.1902) -> (5.5948, -3.1902)
  line L244 (5.5948, -3.1902) -> (5.5948, -1.9899)
  line L245 (5.5948, -1.9899) -> (8.8939, -1.9899)
  line L246 (8.8939, -1.9899) -> (8.8939, -3.1902)
  line L247 (8.8939, -3.1902) -> (10.6192, -3.1902)
  line L248 (10.6192, -3.1902) -> (10.6192, -7.6605)
  line L249 (10.6192, -7.6605) -> (11.344, -7.6605)
  line L250 (11.344, -7.6605) -> (11.344, -3.5609)
  line L251 (11.344, -3.5609) -> (12.1447, -3.5609)
  line L252 (40.7197, -22.6109) -> (40.7197, -21.01)
  line L253 (40.7197, -21.01) -> (54.719, -21.01)
  line L254 (54.719, -21.01) -> (54.719, -22.6109)
  line L255 (54.719, -22.6109) -> (55.5198, -22.6109)
  line L256 (55.5198, -22.6109) -> (55.5198, -35.4101)
  line L257 (55.5198, -35.4101) -> (54.719, -35.4101)
  line L258 (54.719, -35.4101) -> (54.719, -37.0094)
  line L259 (54.719, -37.0094) -> (40.7197, -37.0094)
  line L260 (40.7197, -37.0094) -> (40.7197, -35.4101)
  line L261 (40.7197, -35.4101) -> (39.9189, -35.4101)
  line L262 (39.9189, -35.4101) -> (39.9189, -22.6109)
  line L263 (39.9189, -22.6109) -> (40.7197, -22.6109)
  line L264 (40.7197, -41.6609) -> (40.7197, -40.0602)
  line L265 (40.7197, -40.0602) -> (54.719, -40.0602)
  line L266 (54.719, -40.0602) -> (54.719, -41.6609)
  line L267 (54.719, -41.6609) -> (55.5198, -41.6609)
  line L268 (55.5198, -41.6609) -> (55.5198, -54.4601)
  line L269 (55.5198, -54.4601) -> (54.719, -54.4601)
  line L270 (54.719, -54.4601) -> (54.719, -56.0594)
  line L271 (54.719, -56.0594) -> (40.7197, -56.0594)
  line L272 (40.7197, -56.0594) -> (40.7197, -54.4601)
  line L273 (40.7197, -54.4601) -> (39.9189, -54.4601)
  line L274 (39.9189, -54.4601) -> (39.9189, -41.6609)
  line L275 (39.9189, -41.6609) -> (40.7197, -41.6609)
  line L276 (21.6697, -22.6109) -> (21.6697, -21.01)
  line L277 (21.6697, -21.01) -> (35.669, -21.01)
  line L278 (35.669, -21.01) -> (35.669, -22.6109)
  line L279 (35.669, -22.6109) -> (36.4698, -22.6109)
  line L280 (36.4698, -22.6109) -> (36.4698, -35.4101)
  line L281 (36.4698, -35.4101) -> (35.669, -35.4101)
  line L282 (35.669, -35.4101) -> (35.669, -37.0094)
  line L283 (35.669, -37.0094) -> (21.6697, -37.0094)
  line L284 (21.6697, -37.0094) -> (21.6697, -35.4101)
  line L285 (21.6697, -35.4101) -> (20.869, -35.4101)
  line L286 (20.869, -35.4101) -> (20.869, -22.6109)
  line L287 (20.869, -22.6109) -> (21.6697, -22.6109)
  line L288 (2.6197, -79.7609) -> (2.6197, -78.1602)
  line L289 (2.6197, -78.1602) -> (16.6192, -78.1602)
  line L290 (16.6192, -78.1602) -> (16.6192, -79.7609)
  line L291 (16.6192, -79.7609) -> (17.4198, -79.7609)
  line L292 (17.4198, -79.7609) -> (17.4198, -92.5601)
  line L293 (17.4198, -92.5601) -> (16.6192, -92.5601)
  line L294 (16.6192, -92.5601) -> (16.6192, -94.1594)
  line L295 (16.6192, -94.1594) -> (2.6196, -94.1594)
  line L296 (2.6197, -94.1594) -> (2.6197, -92.5601)
  line L297 (2.6197, -92.5601) -> (1.819, -92.5601)
  line L298 (1.819, -92.5601) -> (1.819, -79.7609)
  line L299 (1.819, -79.7609) -> (2.6197, -79.7609)
  line L300 (40.7197, -3.5609) -> (40.7197, -1.96)
  line L301 (40.7197, -1.96) -> (54.719, -1.96)
  line L302 (54.719, -1.96) -> (54.719, -3.5609)
  line L303 (54.719, -3.5609) -> (55.5198, -3.5609)
  line L304 (55.5198, -3.5609) -> (55.5198, -16.3601)
  line L305 (55.5198, -16.3601) -> (54.719, -16.3601)
  line L306 (54.719, -16.3601) -> (54.719, -17.9595)
  line L307 (54.719, -17.9595) -> (40.7197, -17.9595)
  line L308 (40.7197, -17.9595) -> (40.7197, -16.3601)
  line L309 (40.7197, -16.3601) -> (39.9189, -16.3601)
  line L310 (39.9189, -16.3601) -> (39.9189, -3.5609)
  line L311 (39.9189, -3.5609) -> (40.7197, -3.5609)
  line L312 (76.2953, -0.4341) -> (0.0951, -0.4341)
  line L313 (0.0951, -0.4341) -> (0.0951, -148.071)
  line L314 (0.0951, -148.071) -> (76.2953, -148.071)
  line L315 (76.2953, -148.071) -> (76.2953, -0.4341)
  line L316 (32.09, -19.4986) -> (5.9194, -19.4986)
  line L317 (0.9194, -14.4986) -> (0.9194, -0.4341)
  line L318 (0.9194, -0.4341) -> (37.09, -0.4341)
  line L319 (37.09, -0.4341) -> (37.09, -14.4986)
  line L320 (76.2953, -36.6991) -> (61.902, -36.6991)
  line L321 (56.902, -31.6991) -> (56.902, -6.8092)
  line L322 (61.902, -1.8092) -> (76.2953, -1.8092)
  line L323 (76.2953, -1.8092) -> (76.2953, -36.6991)
  line L324 (76.2953, -75.8337) -> (61.902, -75.8337)
  line L325 (56.902, -70.8337) -> (56.902, -44.1838)
  line L326 (61.902, -39.1838) -> (76.2953, -39.1838)
  line L327 (76.2953, -39.1838) -> (76.2953, -75.8337)
  arc A0 (56.902, -70.8337) -> (61.902, -75.8337) centre (61.902, -70.8337) ccw
  arc A1 (61.902, -39.1838) -> (56.902, -44.1838) centre (61.902, -44.1838) ccw
  arc A2 (56.902, -31.6991) -> (61.902, -36.6991) centre (61.902, -31.6991) ccw
  arc A3 (61.902, -1.8092) -> (56.902, -6.8092) centre (61.902, -6.8092) ccw
  arc A4 (32.09, -19.4986) -> (37.09, -14.4986) centre (32.09, -14.4986) ccw
  arc A5 (0.9194, -14.4986) -> (5.9194, -19.4986) centre (5.9194, -14.4986) ccw
  dimension "d37" = 5
  constraint horizontal L316
  constraint vertical L317
  constraint horizontal L318
  constraint vertical L319
  constraint coincident L312 L317.end
  constraint horizontal L320
  constraint vertical L321
  constraint horizontal L322
  constraint vertical L323
  constraint coincident L315 L320.start
  constraint horizontal L324
  constraint vertical L325
  constraint horizontal L326
  constraint vertical L327
  constraint coincident L315 L324.start
  constraint tangent L324 A0
  constraint tangent L325 A0
  constraint tangent L325 A1
  constraint tangent L326 A1
  constraint equal A0 A1
  constraint tangent L320 A2
  constraint tangent L321 A2
  constraint equal A0 A2
  constraint tangent L321 A3
  constraint tangent L322 A3
  constraint equal A0 A3
  constraint tangent L316 A4
  constraint tangent L319 A4
  constraint equal A0 A4
  constraint tangent L316 A5
  constraint tangent L317 A5
  constraint equal A0 A5
  measures "d37" radius of A0
extrude "Extrude18" cut sketch "Sketch2" against normal blind 40 contours L312 L316 L317 L318 L319 A4 A5 | L315 L320 L321 L322 L323 A2 A3 | L315 L324 L325 L326 L327 A0 A1 bodies 2